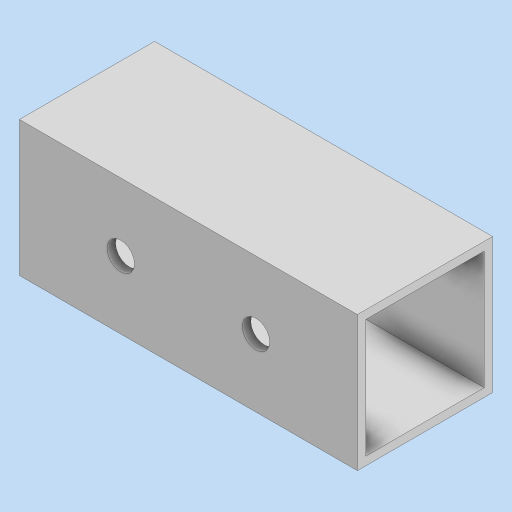
# Autodesk Inventor part: 1inTubeBase
Saved by Autodesk Inventor 2024 (Build 280153000, 153)
## iProperties
Created: 2024-01-10
Part Number: 1inTubeBase
Material: Generic
Document SubType Name: Modeling
Designer: megan
Density: 1 g/cm^3
Appearance: Default
Author: megan
Autodesk Inventor part; units mm, degrees
ref_plane "YZ Plane" through (0, 0, 0) normal (1, 0, 0) x (0, 1, 0)
ref_plane "XZ Plane" through (0, 0, 0) normal (0, 1, 0) x (-1, 0, 0)
ref_plane "XY Plane" through (0, 0, 0) normal (0, 0, 1) x (1, 0, 0)
sketch "Sketch1" plane through (0, 0, 0) normal (1, 0, 0) x (0, 1, 0)
  line L0 (0, 0) -> (25.4, 0)
  line L1 (25.4, 0) -> (25.4, -25.4)
  line L2 (25.4, -25.4) -> (0, -25.4)
  line L3 (0, -25.4) -> (0, 0)
  line L4 (23.8125, -23.8125) -> (23.8125, -1.5875)
  line L5 (23.8125, -1.5875) -> (1.5875, -1.5875)
  line L6 (1.5875, -1.5875) -> (1.5875, -23.8125)
  line L7 (1.5875, -23.8125) -> (23.8125, -23.8125)
  dimension "d0" = 25.4
  dimension "d1" = 25.4
  dimension "d2" = 1.5875
  constraints: 16 end point, 4 parallel, 2 perpendicular, 1 horizontal, 3 other
  measures "d0" distance of L1.end L2.end
  measures "d1" distance of L0.end L1.end
  measures "d2" distance between parallel lines of L1 L4
extrude "Extrusion1" add sketch "Sketch1" along normal mid plane 63.5
sketch "Sketch3" plane through (-31.75, 0, 0) normal (0, 0, 1) x (1, 0, 0)
  line L0 (0, 0) -> (63.5, 0) projected
  line L1 (63.5, 25.4) -> (63.5, 0) projected
  line L2 (0, 25.4) -> (63.5, 25.4) projected
  line L3 (0, 0) -> (0, 25.4) projected
  circle A0 centre (19.05, 12.7) radius 2.5781
  circle A1 centre (44.45, 12.7) radius 2.5781
  line L4 (31.75, 25.4) -> (31.75, 0) construction
  dimension "d14" = 5.1562
  dimension "d15" = 5.1562
  dimension "d16" = 12.7
  dimension "d17" = 25.4
  dimension "d20" = 12.7
  constraints: 2 centre point, 2 end point, 1 horizontal alignment, 1 midpoint, 1 vertical
  measures "d14" diameter of A0
  measures "d15" diameter of A1
  measures "d16" distance from line of L4 A0.centre
  measures "d17" distance of A1.centre A0.centre
  measures "d20" distance from line of L2 A0.centre
extrude "Extrusion3" cut sketch "Sketch3" against normal blind 25.4 contours A0 | A1
body "Solid1"
